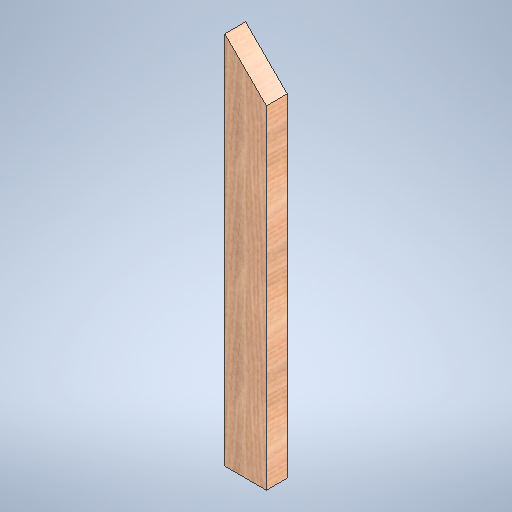
# Autodesk Inventor part: 2x4x36 (45 90)
Saved by Autodesk Inventor 2025 (Build 290162000, 162)
## iProperties
Created: 2024-07-01
Part Number: 2x4x36 (45 90)
Material: Generic
Document SubType Name: Modeling
Designer: Cupri
Density: 1 g/cm^3
Appearance: Default
Author: Cupri
Autodesk Inventor part; units mm, degrees
ref_plane "YZ Plane" through (0, 0, 0) normal (1, 0, 0) x (0, 1, 0)
ref_plane "XZ Plane" through (0, 0, 0) normal (0, 1, 0) x (-1, 0, 0)
ref_plane "XY Plane" through (0, 0, 0) normal (0, 0, 1) x (1, 0, 0)
sketch "Sketch1" plane through (0, 0, 0) normal (0, 0, 1) x (1, 0, 0)
  line L0 (0, 0) -> (101.6, 0)
  line L1 (101.6, 0) -> (101.6, 812.8)
  line L2 (0, 914.4) -> (0, 0)
  line L3 (0, 914.4) -> (101.6, 812.8)
  dimension "d1" = 914.4
  constraints: 8 end point, 1 horizontal, 1 parallel, 1 perpendicular
  measures "d1" distance of L2.start L0.start
extrude "Extrusion1" add sketch "Sketch1" along normal blind 50.8
body "Solid1"
